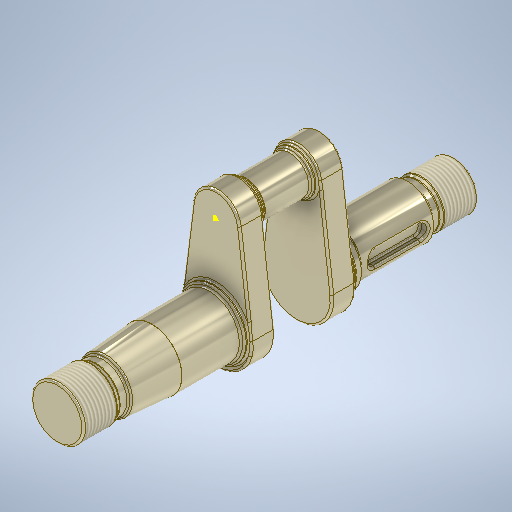
# Autodesk Inventor part: Crankshaft
Saved by Autodesk Inventor 2025.1 (Build 291241000, 241)
## iProperties
Created: 2024-07-27
Part Number: Crankshaft
Material: Iron, Cast
Document SubType Name: Modeling
Designer: vedan
Density: 7.15 g/cm^3
Appearance: Nickel
Author: vedan
Autodesk Inventor part; units mm, degrees
sketch "Sketch1" plane through (0, 0, 0) normal (0, 1, 0) x (-1, 0, 0)
  point P0 (0, 0)
sketch "Sketch2" plane through (0, 0, 0) normal (0, 0, 1) x (1, 0, 0)
  point P0 (0, 0)
sketch "Sketch3" plane through (0, 0, 0) normal (0, 0, 1) x (1, 0, 0)
  arc A0 (9.9216, 1.25) -> (-9.9216, 1.25) centre (0, 0) ccw
  line L0 (0, 0) -> (0, -40) construction
  arc A1 (-14.8824, -38.125) -> (14.8824, -38.125) centre (0, -40) ccw
  line L1 (-14.8824, -38.125) -> (-9.9216, 1.25)
  line L2 (14.8824, -38.125) -> (9.9216, 1.25)
  dimension "d2" = 40
  dimension "d3" = 30
  constraints: 6 end point, 4 point on circle, 4 tangent, 2 centre point, 2 coincident, 1 vertical
  measures "d2" distance of L0.start L0.end
  measures "d3" diameter of A1
extrude "Extrusion1" add sketch "Sketch3" against normal blind 10
sketch "Sketch4" plane through (0, 0, -10) normal (0, 0, -1) x (-1, 0, 0)
  circle A0 centre (0, 0) radius 9
  dimension "d6" = 18
  constraints: 1 centre point, 1 coincident
  measures "d6" diameter of A0
extrude "Extrusion2" add sketch "Sketch4" along normal blind 2
sketch "Sketch5" plane through (0, 0, -12) normal (0, 0, -1) x (-1, 0, 0)
  circle A0 centre (0, 0) radius 8
  dimension "d9" = 16
  constraints: 1 centre point, 1 coincident
  measures "d9" diameter of A0
extrude "Extrusion3" add sketch "Sketch5" along normal blind 10
ref_plane "Work Plane1" through (0, 0, -22) normal (0, 0, 1) x (1, 0, 0)
mirror "Mirror1" about plane through (0, 0, -22) normal (0, 0, 1) of "Extrusion1", "Extrusion2", "Extrusion3"
sketch "Sketch6" plane through (0, 0, 0) normal (0, 0, 1) x (1, 0, 0)
  point P0 (0, 0)
sketch "Sketch7" plane through (0, 0, 0) normal (0, 0, 1) x (1, 0, 0)
  point P0 (0, 0)
sketch "Sketch8" plane through (14.8824, -38.125, 0) normal (0.9921567, 0.125, 0) x (0, 0, -1)
  point P0 (0, 39.6863)
sketch "Sketch9" plane through (0, 0, -10) normal (0, 0, -1) x (-1, 0, 0)
  point P0 (0, 0)
sketch "Sketch10" plane through (0, 0, 0) normal (0, 0, 1) x (1, 0, 0)
  point P0 (0, 0)
sketch "Sketch11" plane through (0, 0, 0) normal (1, 0, 0) x (0, 1, 0)
  line L0 (-38.125, 0) -> (-38.125, 67)
  line L1 (-38.125, 0) -> (-24.125, 0)
  line L2 (1.25, 0) -> (-38.125, 0) projected
  line L3 (-24.125, 0) -> (-24.125, 2)
  line L4 (-24.125, 2) -> (-38.125, 2)
  line L5 (-24.125, 2) -> (-25.4701, 2)
  line L6 (-25.4701, 2) -> (-25.4701, 27)
  line L7 (-25.4701, 27) -> (-38.125, 27)
  line L8 (-25.4701, 27) -> (-26.9579, 47)
  line L9 (-26.9579, 47) -> (-38.125, 47)
  line L10 (-26.9579, 47) -> (-27.9579, 47)
  line L11 (-26.9579, 47) -> (-26.9579, 27) construction
  line L12 (-26.9579, 47) -> (-27.6881, 47)
  line L13 (-27.9579, 47) -> (-27.9579, 50.7758)
  line L14 (-27.9579, 50.7758) -> (-26.9579, 52.7954)
  line L15 (-26.9579, 52.7954) -> (-26.9579, 67)
  line L16 (-26.9579, 67) -> (-38.125, 67)
  line L17 (-26.9579, 67) -> (-26.9579, 47) construction
  point P0 (0, 0)
  point P1 (-27.4579, 47)
  dimension "d14" = 67
  dimension "d15" = 14
  dimension "d17" = 2
  dimension "d20" = 25
  dimension "d21" = 20
  dimension "d22" = 1
  dimension "d23" = 20
  constraints: 34 end point, 9 point on line, 6 vertical, 2 horizontal, 2 perpendicular, 1 midpoint, 1 parallel
  measures "d14" distance of L0.start L0.end
  measures "d15" distance of L0.start L1.end
  measures "d17" distance of L1.end L3.end
  measures "d20" distance of L5.end L6.end
  measures "d21" distance of L8.end L11.end
  measures "d22" distance of L10.end L8.end
  measures "d23" vertical distance of point (-27.458, 47) L15.end
revolve "Revolution1" add sketch "Sketch11" angle 360 about axis through (0, -38.125, 0) along (0, 0, 1)
sketch "Sketch12" plane through (9.9216, 1.25, -34) normal (0.9921567, 0.125, 0) x (0, 0, -1)
  point P0 (-34, 0)
sketch "Sketch13" plane through (0, -40, -44) normal (0, 0, -1) x (-1, 0, 0)
  point P0 (0, 40)
sketch "Sketch14" plane through (0, 0, 0) normal (1, 0, 0) x (0, 1, 0)
  line L0 (-38.125, 0) -> (-55, 0) construction
  line L1 (-38.125, -44) -> (-38.125, -34) construction
  line L2 (-38.125, 0) -> (-38.125, -44) construction
  line L3 (-38.125, -44) -> (-24.125, -44)
  line L4 (1.25, -44) -> (-38.125, -44) projected
  line L5 (-24.125, -44) -> (-24.125, -46)
  line L6 (-24.125, -46) -> (-25.625, -46)
  line L7 (-25.625, -46) -> (-25.625, -49.6748)
  line L8 (-25.625, -49.6748) -> (-27.125, -49.6748)
  line L9 (-27.125, -49.6748) -> (-27.125, -81.6748)
  line L10 (-27.125, -81.6748) -> (-28.8475, -81.6748)
  line L11 (-38.125, -44) -> (-38.125, -100.7747)
  line L12 (-25.625, -46) -> (-38.125, -46)
  line L13 (-27.125, -49.6748) -> (-38.125, -49.6748)
  line L14 (-38.125, -53.6748) -> (-38.125, -78.4772) construction
  line L15 (-27.125, -81.6748) -> (-38.125, -81.6748)
  line L16 (-30.1345, -101.6748) -> (-30.1345, -49.6748) construction
  line L17 (-32.4024, -81.6748) -> (-32.4024, -101.6748) construction
  line L18 (-38.125, -81.6748) -> (-28.8475, -81.6748)
  line L19 (-28.8475, -81.6748) -> (-28.8475, -85.0351)
  line L20 (-28.8475, -85.0351) -> (-28.125, -86.3818)
  line L21 (-28.125, -86.3818) -> (-28.125, -100.7747)
  line L22 (-28.125, -100.7747) -> (-38.125, -100.7747)
  line L23 (-28.125, -100.7747) -> (-28.8475, -101.6748)
  line L24 (-28.8475, -101.6748) -> (-37.0037, -101.6748)
  line L25 (-37.0037, -101.6748) -> (-38.125, -100.7747)
  line L26 (-28.125, -86.3818) -> (-38.125, -86.3818)
  point P0 (0, 0)
  dimension "d42" = 2
  dimension "d80" = 14
  dimension "d81" = 12.5
  dimension "d82" = 1.5
  dimension "d83" = 1.5
  dimension "d84" = 52
  dimension "d85" = 20
  dimension "d89" = 11
  dimension "d90" = 10
  constraints: 50 end point, 10 perpendicular, 9 point on line, 4 vertical, 2 parallel, 1 collinear, 1 horizontal
  measures "d42" distance of L5.end L3.end
  measures "d80" distance from line of L1 L3.end
  measures "d81" distance of L12.end L6.end
  measures "d82" distance of L8.end L7.end
  measures "d83" distance of L6.end L5.end
  measures "d84" distance of L16.start L16.end
  measures "d85" distance of L17.start L17.end
  measures "d89" distance of L15.end L9.end
  measures "d90" distance of L26.end L20.end
revolve "Revolution2" add sketch "Sketch14" angle 360 about axis through (0, -38.125, -44) along (0, 0, -1) contours L3 L5 L6 L12 L11 | L12 L7 L8 L13 L11 | L13 L9 L10 L15 L11 | L15 L19 L20 L26 L11 | L26 L21 L22 L11
sketch "Sketch15" plane through (0, 0, 0) normal (1, 0, 0) x (0, 1, 0)
  point P0 (0, 0)
  point P1 (-38.1229, -63.8655)
ref_plane "Work Plane7" through (11, 0, 0) normal (1, 0, 0) x (0, 1, 0)
sketch "Sketch24" plane through (11, 0, 0) normal (1, 0, 0) x (0, 1, 0)
  line L0 (-49.125, -49.6748) -> (-27.125, -49.6748) projected
  line L1 (-38.125, -53.6748) -> (-38.125, -78.6748) construction
  point P0 (0, 0)
  point P1 (-38.125, -66.1748)
  constraints: 4 end point, 1 midpoint, 1 vertical
ref_plane "Work Plane9" through (11, 0, 0) normal (1, 0, 0) x (0, 1, 0)
sketch "Sketch28" plane through (11, 0, 0) normal (1, 0, 0) x (0, 1, 0)
  line L0 (-50.625, -49.6748) -> (-25.625, -49.6748) construction
  line L1 (-38.125, -49.6748) -> (-38.125, -53.6748) construction
  line L2 (-38.125, -53.6748) -> (-38.125, -78.6748) construction
  line L3 (-41.125, -56.6748) -> (-41.125, -75.6748)
  line L4 (-35.125, -75.6748) -> (-35.125, -56.6748)
  arc A0 (-35.125, -56.6748) -> (-41.125, -56.6748) centre (-38.125, -56.6748) ccw
  arc A1 (-41.125, -75.6748) -> (-35.125, -75.6748) centre (-38.125, -75.6748) ccw
  point P0 (0, 0)
  point P1 (-38.125, -66.1748)
  dimension "d92" = 4
  dimension "d93" = 25
  constraints: 10 end point, 6 point on circle, 4 tangent, 2 centre point, 2 midpoint, 2 point on line, 2 vertical, 1 parallel
  measures "d92" distance of L1.start L1.end
  measures "d93" distance of L1.end L2.end
sketch "Sketch29" plane through (11, 0, 0) normal (1, 0, 0) x (0, 1, 0)
  point P0 (0, 0)
extrude "Extrusion7" cut sketch "Sketch28" against normal blind 3.5
fillet "Fillet1" radius 0.8 17 edges at (8, 0, -32) (8, 0, -12) (9, 0, -34) (9, 0, -10) (0, -52.125, -44) (0, -52.125, 0) (0, -50.625, -46) (0, -50.7799, 2) (0, -49.125, -49.6748) (0, -47.4025, -81.6748) (7.5, -41.125, -66.1748) (7.5, -38.125, -53.6748) (7.5, -35.125, -66.1748) (7.5, -38.125, -78.6748) (0, -48.2921, 47) (0, -47.4025, -85.0351) (0, -48.2921, 50.7758)
fillet "Fillet1" radius 0.8 33 edges at (9, 0, -32) (9, 0, -12) (0, -55, -34) (-12.402, -18.4375, -34) (12.402, -18.4375, -34) (0, 10, -34) (0, -55, -44) (-12.402, -18.4375, -44) (12.402, -18.4375, -44) (0, 10, -44) (0, -55, -10) (-12.402, -18.4375, -10) (12.402, -18.4375, -10) (0, 10, -10) (0, -55, 0) (-12.402, -18.4375, 0) (12.402, -18.4375, 0) (0, 10, 0) (0, -52.125, -46) (0, -52.125, 2) (0, -50.625, -49.6748) (0, -49.125, -81.6748) (10.583, -41.125, -66.1748) (10.761, -40.4057, -54.7258) (10.7614, -35.8465, -54.7233) (10.583, -35.125, -66.1748) (10.7618, -35.8483, -77.6284) (10.761, -40.4056, -77.6239) (0, -49.2921, 47) (0, -48.125, -86.3818) (0, -49.2921, 52.7954) (0, -48.125, -100.7747) (0, -49.2921, 67)
thread "Thread1" size "M20x1.5" class "6g" standard "ANSI Metric M Profile" full length
thread "Thread2" size "M20x1.5" class "6g" standard "ANSI Metric M Profile" full length
sketch "Sketch30" plane through (0, 0, 0) normal (1, 0, 0) x (0, 1, 0)
  point P0 (0, 0)
body "Solid1"
